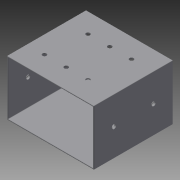
# Autodesk Inventor part: Box Base
Saved by Autodesk Inventor 2014 (Build 180170000, 170)
## iProperties
Created: 2014-05-19
Part Number: Box Base
Material: Generic
Document SubType Name: Modeling
Designer: lpluta-ehlers
Density: 1 g/cm^3
Appearance: Default
Author: lpluta-ehlers
Autodesk Inventor part; units mm, degrees
ref_plane "YZ Plane" through (0, 0, 0) normal (1, 0, 0) x (0, 1, 0)
ref_plane "XZ Plane" through (0, 0, 0) normal (0, 1, 0) x (-1, 0, 0)
ref_plane "XY Plane" through (0, 0, 0) normal (0, 0, 1) x (1, 0, 0)
sketch "Sketch1" plane through (0, 0, 0) normal (0, 1, 0) x (-1, 0, 0)
  line L0 (0, 0) -> (-279.4, 0)
  line L1 (-279.4, 0) -> (-279.4, -254)
  line L2 (-279.4, -254) -> (0, -254)
  line L3 (0, -254) -> (0, 0)
  dimension "blength" = 279.4
  dimension "bwidth" = 254
  constraints: 8 end point, 2 parallel, 1 horizontal, 1 perpendicular
  measures "blength" distance of L1.end L2.end
  measures "bwidth" distance of L0.end L1.end
extrude "Extrusion1" add sketch "Sketch1" along normal blind 177.8
shell "Shell1" thickness 3.81 removed faces 2 at (93.1333, 118.5333, 0) at (186.2667, 59.2667, -254)
sketch "Sketch2" plane through (279.4, 0, 0) normal (1, 0, 0) x (0, 0, -1)
  line L0 (0, 0) -> (254, 0) projected
  line L1 (254, 0) -> (254, 177.8) projected
  line L2 (0, 177.8) -> (254, 177.8) projected
  line L3 (0, 0) -> (0, 177.8) projected
  circle A0 centre (63.5, 88.9) radius 6.35
  circle A1 centre (190.5, 88.9) radius 6.35
  line L4 (127, 177.8) -> (127, 0) construction
  line L5 (63.5, 177.8) -> (63.5, 50.8) construction
  line L6 (190.5, 177.8) -> (190.5, 50.8) construction
  line L7 (0, 88.9) -> (254, 88.9) construction
  dimension "csize" = 12.7
  dimension "d6" = 12.7
  dimension "sidecirclemasterxloc" = 127
  dimension "sidecirclexloc" = 63.5
  dimension "sidecircle2xloc" = 63.5
  dimension "sidecircleyloc" = 88.9
  dimension "d11" = 0
  dimension "d12" = 127
  dimension "d13" = 0
  dimension "d14" = 127
  constraints: 8 end point, 4 midpoint, 4 point on line, 2 centre point, 2 parallel, 2 perpendicular
  measures "csize" diameter of A0
  measures "d6" diameter of A1
  measures "sidecirclemasterxloc" distance between parallel lines of L1 L4
  measures "sidecirclexloc" distance between parallel lines of L5 L4
  measures "sidecircle2xloc" distance between parallel lines of L6 L4
  measures "sidecircleyloc" distance between parallel lines of L2 L7
  measures "d11" distance from line of L6.start L2
  measures "d12" distance from line of L6.end L2
  measures "d13" distance from line of L5.start L2
  measures "d14" distance from line of L5.end L2
extrude "Extrusion2" cut sketch "Sketch2" against normal blind 304.8 contours A0 | A1
sketch "Sketch3" plane through (0, 177.8, 0) normal (0, 1, 0) x (1, 0, 0)
  line L0 (22.225, 190.5) -> (212.725, 190.5) construction
  circle A0 centre (45.72, 190.5) radius 6.35
  circle A1 centre (147.32, 190.5) radius 6.35
  circle A2 centre (242.57, 190.5) radius 6.35
  circle A3 centre (64.55, 63.5) radius 6.35
  circle A4 centre (140.75, 63.5) radius 6.35
  circle A5 centre (223.3, 63.5) radius 6.35
  line L1 (0, 0) -> (279.4, 0) projected
  line L2 (279.4, 0) -> (279.4, 254) projected
  line L3 (0, 0) -> (279.4, 0) construction
  line L4 (45.72, 557.1547) -> (45.72, -109.5361)
  line L5 (242.57, 131.8408) -> (242.57, 276.0016)
  line L6 (147.32, 557.1547) -> (147.32, -109.5361)
  line L7 (223.3, 557.1547) -> (223.3, -109.5361)
  line L8 (140.75, 127.0264) -> (140.75, -37.848)
  line L9 (64.55, 557.1547) -> (64.55, -109.5361)
  dimension "d22" = 12.7
  dimension "d23" = 12.7
  dimension "d24" = 12.7
  dimension "d28" = 12.7
  dimension "d29" = 12.7
  dimension "d30" = 12.7
  dimension "d57" = 66.675
  dimension "d71" = 257.175
  dimension "d74" = 0
  dimension "d75" = 0
  dimension "d76" = 0
  dimension "d77" = 0
  dimension "d78" = 0
  dimension "d79" = 0
  constraints: 16 end point, 6 centre point, 6 vertical, 3 point on line, 1 collinear, 12 other
  measures "d22" diameter of A0
  measures "d23" diameter of A1
  measures "d24" diameter of A2
  measures "d28" diameter of A3
  measures "d29" diameter of A4
  measures "d30" diameter of A5
  measures "d57" distance from line of L0.end L2
  measures "d71" distance from line of L0.start L2
  measures "d74" distance from line of L4 A0.centre
  measures "d75" distance from line of L6 A1.centre
  measures "d76" distance from line of A2.centre L5
  measures "d77" distance from line of L9 A3.centre
  measures "d78" distance from line of L8 A4.centre
  measures "d79" distance from line of A5.centre L7
extrude "Extrusion3" cut sketch "Sketch3" against normal blind 50.8
sketch "Sketch7" plane through (279.4, 0, 0) normal (1, 0, 0) x (0, 0, -1)
  circle A0 centre (63.5, 88.9) radius 6.35 projected
  circle A1 centre (190.5, 88.9) radius 6.35 projected
  circle A2 centre (63.5, 88.9) radius 6.477
  circle A3 centre (190.5, 88.9) radius 6.477
  dimension "cholder" = 12.954
  dimension "d39" = 12.954
  constraints: 2 centre point, 2 coincident
  measures "cholder" diameter of A2
  measures "d39" diameter of A3
extrude "Extrusion4" add sketch "Sketch7" along normal blind 1.27 and the other way blind 5.08
sketch "Sketch8" plane through (0, 0, -254) normal (-1, 0, 0) x (0, 0, 1)
  circle A0 centre (190.5, 88.9) radius 6.35 projected
  circle A1 centre (63.5, 88.9) radius 6.35 projected
  circle A2 centre (63.5, 88.9) radius 6.477
  circle A3 centre (190.5, 88.9) radius 6.477
  dimension "d44" = 12.954
  dimension "d45" = 12.954
  constraints: 2 centre point, 2 coincident
  measures "d44" diameter of A2
  measures "d45" diameter of A3
extrude "Extrusion5" add sketch "Sketch8" along normal blind 1.27 and the other way blind 5.08
fillet "Fillet1" radius 1.27 24 edges at (0, 177.8, -127) (139.7, 177.8, -254) (279.4, 177.8, -127) (139.7, 177.8, 0) (0, 88.9, -254) (3.81, 88.9, -254) (139.7, 173.99, -254) (275.59, 88.9, -254) (279.4, 88.9, -254) (139.7, 3.81, -254) (139.7, 0, -254) (275.59, 3.81, -127) (3.81, 88.9, 0) (0, 88.9, 0) (0, 0, -127) (3.81, 3.81, -127) (275.59, 88.9, 0) (139.7, 173.99, 0) (139.7, 3.81, 0) (139.7, 0, 0) (279.4, 88.9, 0) (279.4, 0, -127) (3.81, 173.99, -127) (275.59, 173.99, -127)
fillet "Fillet2" radius 0.254 20 edges at (216.95, 177.8, -63.5) (134.4, 177.8, -63.5) (58.2, 177.8, -63.5) (39.37, 177.8, -190.5) (140.97, 177.8, -190.5) (236.22, 177.8, -190.5) (216.95, 173.99, -63.5) (134.4, 173.99, -63.5) (39.37, 173.99, -190.5) (140.97, 173.99, -190.5) (236.22, 173.99, -190.5) (58.2, 173.99, -63.5) (280.67, 88.9, -57.15) (280.67, 88.9, -184.15) (-1.27, 88.9, -69.85) (-1.27, 88.9, -196.85) (274.32, 88.9, -57.15) (5.08, 88.9, -69.85) (5.08, 88.9, -196.85) (274.32, 88.9, -184.15)
equation "\"d6\" = csize"
equation "\"sidecirclexloc\" = topCircDistFromCntr"
equation "\"sidecircle2xloc\" = sidecirclexloc"
equation "\"sidecircleyloc\" = 0.5 * bheight"
equation "\"d22\" = csize"
equation "\"d23\" = csize"
equation "\"d24\" = csize"
equation "\"d28\" = csize"
equation "\"d29\" = csize"
equation "\"d30\" = csize"
equation "\"d39\" = cholder"
equation "\"d44\" = cholder"
equation "\"d45\" = cholder"
equation "\"d46\" = sideExtrusionOUT"
equation "\"d47\" = sideExtrusionIN"
equation "\"topCircDistFromCntr\" = 0.25 * bwidth"
equation "\"bheight\" = 177.8"
equation "\"sideExtrusionOUT\" = 1.27"
equation "\"sideExtrusionIN\" = 5.08"
body "Solid1"
